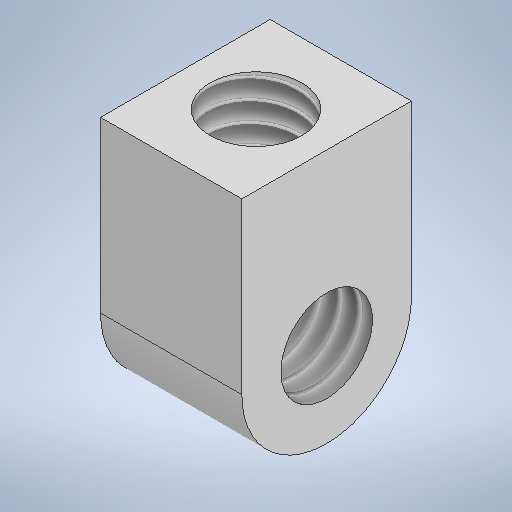
# Autodesk Inventor part: CONECTOR U-L
Saved by Autodesk Inventor 2025.2 (Build 292293000, 293)
## iProperties
Created: 2025-05-14
Part Number: CONECTOR U-L
Material: Genérico
Document SubType Name: Modeling
Designer: marce
Density: 1 g/cm^3
Appearance: Padrão
Author: marce
Autodesk Inventor part; units mm, degrees
ref_plane "YZ Plane" through (0, 0, 0) normal (1, 0, 0) x (0, 1, 0)
ref_plane "XZ Plane" through (0, 0, 0) normal (0, 1, 0) x (-1, 0, 0)
ref_plane "XY Plane" through (0, 0, 0) normal (0, 0, 1) x (1, 0, 0)
sketch "Esboço1" plane through (0, 0, 0) normal (1, 0, 0) x (0, 1, 0)
  line L0 (0, 0) -> (5.9987, 0)
  line L1 (5.9987, 0) -> (5.9987, -6)
  line L2 (5.9987, -6) -> (-0.0013, -6)
  arc A0 (0, 0) -> (-0.0013, -6) centre (-0.0007, -3) ccw
  dimension "d0" = 6
  dimension "d1" = 6
  dimension "d3" = 3
  constraints: 6 end point, 2 perpendicular, 2 point on circle, 1 centre point, 1 horizontal
  measures "d0" distance of L0.end L1.end
  measures "d1" distance of L1.end L2.end
  measures "d3" radius of A0
extrude "Extrusão1" add sketch "Esboço1" along normal blind 5
sketch "Esboço2" plane through (5, 0, 0) normal (1, 0, 0) x (0, 0, -1)
  arc A0 (0, 0) -> (6, -0.0013) centre (3, -0.0007) ccw projected
  constraints: 1 coincident
hole "Furo1" at (5, -0.0007, -3) direction (-1, 0, 0) diameter 3.242 depth 4 thread size "M4x0.7" class "6H" standard "ANSI Metric M Profile"
sketch "Esboço3" plane through (0, 5.9987, 0) normal (0, 1, 0) x (1, 0, 0)
  line L0 (5, 0) -> (5, 6) projected
  line L1 (0, 6) -> (0, 0) projected
  point P0 (2.5, 3)
hole "Furo2" at (2.5, 5.9987, -3) direction (0, -1, 0) diameter 3.242 depth 4 thread size "M4x0.7" class "6H" standard "ANSI Metric M Profile"
